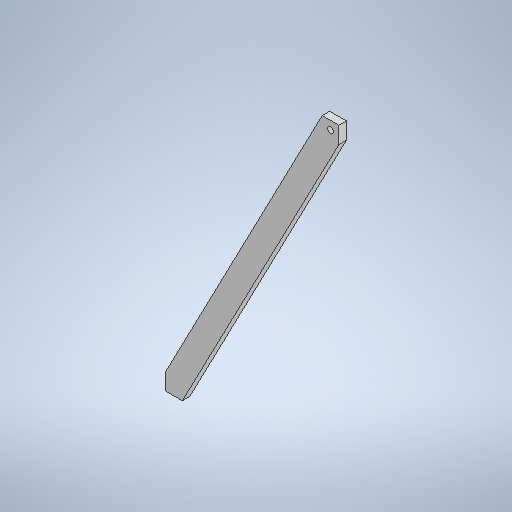
# Autodesk Inventor part: Support - Left
Saved by Autodesk Inventor 2025.2 (Build 292293000, 293)
## iProperties
Created: 2025-02-17
Part Number: Support - Left
Material: Generic
Document SubType Name: Modeling
Designer: baolo
Density: 1 g/cm^3
Appearance: Default
Author: baolo
Autodesk Inventor part; units mm, degrees
ref_plane "YZ Plane" through (0, 0, 0) normal (1, 0, 0) x (0, 1, 0)
ref_plane "XZ Plane" through (0, 0, 0) normal (0, 1, 0) x (-1, 0, 0)
ref_plane "XY Plane" through (0, 0, 0) normal (0, 0, 1) x (1, 0, 0)
sketch "Sketch1" plane through (0, 0, 0) normal (0, 0, 1) x (1, 0, 0)
  line L0 (0, 22.2362) -> (22.2362, 22.2362) construction
  line L1 (22.2362, 22.2362) -> (22.2362, 0) construction
  line L2 (22.2362, 0) -> (0, 0)
  line L3 (0, 0) -> (0, 22.2362)
  line L4 (0, 22.2362) -> (22.2362, 0) construction
  line L5 (22.2362, 22.2362) -> (0, 0) construction
  line L6 (208.1103, 421.1181) -> (230.3465, 421.1181)
  line L7 (230.3465, 421.1181) -> (230.3465, 398.8819)
  line L8 (230.3465, 398.8819) -> (208.1103, 398.8819) construction
  line L9 (208.1103, 398.8819) -> (208.1103, 421.1181) construction
  line L10 (208.1103, 421.1181) -> (230.3465, 398.8819) construction
  line L11 (230.3465, 421.1181) -> (208.1103, 398.8819) construction
  line L12 (208.1103, 421.1181) -> (0, 22.2362)
  line L13 (230.3465, 398.8819) -> (22.2362, 0)
  line L14 (0, 0) -> (230.3465, 421.1181) construction
  line L15 (-46.0693, 0) -> (276.4159, 0) construction
  point P0 (11.1181, 11.1181)
  point P1 (219.2284, 410)
  point P2 (115.1733, 210.5591)
  dimension "d1" = 480
  dimension "d14" = 410
  dimension "d15" = 30
  constraints: 30 end point, 5 midpoint, 4 parallel, 3 equal length, 2 horizontal, 2 perpendicular, 1 coincident
  measures "d1" distance of L2.end L6.end
  measures "d14" distance from line of L15 point (219.228, 410)
  measures "d15" distance between parallel lines of L13 L12
extrude "Extrusion1" add sketch "Sketch1" along normal mid plane 10
sketch "Sketch2" plane through (0, 0, 5) normal (0, 0, 1) x (1, 0, 0)
  line L0 (230.3465, 421.1181) -> (208.1103, 421.1181) construction
  line L1 (230.3465, 398.8819) -> (230.3465, 421.1181) construction
  line L2 (208.1103, 421.1181) -> (230.3465, 398.8819) construction
  point P0 (0, 0)
  point P1 (219.2284, 410)
  constraints: 2 end point, 1 midpoint
hole "Hole1" at (219.2284, 410, 5) direction (0, 0, -1) diameter 8 end through all
body "Solid1"
